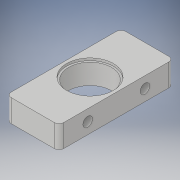
# Autodesk Inventor part: BearingBlock30mmLeft
Saved by Autodesk Inventor 2018 (Build 220112000, 112)
## iProperties
Created: 2017-11-02
Part Number: BearingBlock30mmLeft
Material: Generic
Document SubType Name: Modeling
Designer: snipe
Density: 1 g/cm^3
Appearance: Default
Author: snipe
Autodesk Inventor part; units mm, degrees
ref_plane "YZ Plane" through (0, 0, 0) normal (1, 0, 0) x (0, 1, 0)
ref_plane "XZ Plane" through (0, 0, 0) normal (0, 1, 0) x (-1, 0, 0)
ref_plane "XY Plane" through (0, 0, 0) normal (0, 0, 1) x (1, 0, 0)
sketch "Sketch1" plane through (0, 0, 0) normal (0, 1, 0) x (-1, 0, 0)
  line L0 (0, -53.34) -> (0, 53.34) projected
  line L1 (-24.5, 0) -> (24.5, 0) projected
  line L2 (24.5, 0) -> (-24.5, 0) projected
  line L3 (0, -53.34) -> (0, 53.34) projected
  line L4 (-17.5, 38.1) -> (-17.5, -38.1)
  line L5 (-17.5, -38.1) -> (17.5, -38.1)
  line L6 (17.5, -38.1) -> (17.5, 38.1)
  line L7 (17.5, 38.1) -> (-17.5, 38.1)
  line L8 (-17.5, -38.1) -> (17.5, 38.1) construction
  point P0 (0, 0)
  dimension "d1" = 76.2
  dimension "d2" = 35
  constraints: 10 end point, 2 parallel, 1 perpendicular, 1 vertical, 2 other
  measures "d1" distance of L4.start L4.end
  measures "d2" distance of L5.end L4.end
extrude "Extrusion1" add sketch "Sketch1" along normal mid plane 15
sketch "Sketch2" plane through (0, 7.5, 0) normal (0, 1, 0) x (1, 0, 0)
  point P0 (0, 0)
  point P1 (0, 0)
  constraints: 1 coincident
hole "Hole1" at (0, 7.5, 0) direction (0, -1, 0) diameter 28.575 end through all counterbore diameter 31.12 counterbore depth 1.588
fillet "Fillet1" radius 3.175 4 edges at (17.5, 0, 38.1) (17.5, 0, -38.1) (-17.5, 0, 38.1) (-17.5, 0, -38.1)
sketch "Sketch3" plane through (-17.5, -7.5, -34.925) normal (-1, 0, 0) x (0, 0, 1)
  line L0 (0, 0) -> (0, 15) projected
  line L1 (69.85, 0) -> (0, 0) projected
  line L2 (69.85, 15) -> (69.85, 0) projected
  line L3 (0, 15) -> (69.85, 15) projected
  line L4 (0, 15) -> (0, 0) projected
  line L5 (0, 0) -> (69.85, 0)
  line L6 (69.85, 0) -> (69.85, 15)
  line L7 (69.85, 15) -> (0, 15)
  line L8 (0, 15) -> (0, 0)
  line L9 (19.365, 15) -> (50.485, 15) projected
  line L10 (34.925, 15) -> (34.925, 0)
  line L11 (0, 7.5) -> (69.85, 7.5)
  line L12 (69.85, 0) -> (69.85, 15) projected
  point P0 (34.925, 7.5)
  point P1 (15.875, 7.5)
  point P2 (53.975, 7.5)
  dimension "d19" = 19.05
  dimension "d20" = 19.05
  constraints: 12 end point, 4 midpoint, 2 parallel, 2 point on line, 1 horizontal, 1 perpendicular
  measures "d19" distance from line of L10 point (15.875, 7.5)
  measures "d20" distance from line of point (53.975, 7.5) L10
hole "Hole2" at (-17.5, 0, -19.05) at (-17.5, 0, 19.05) direction (1, 0, 0) diameter 6.35 end through all counterbore diameter 9.525 counterbore depth 6.35
body "Solid1"
